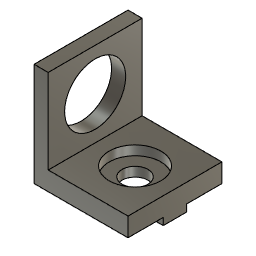
cable_holder (Autodesk Fusion 360 design; units mm, degrees)
Autodesk Fusion 360 part; units mm, degrees
sketch "Sketch1" plane through (0, 0, 0) normal (0, 0, 1) x (1, 0, 0)
  line L0 (0, 0) -> (20, 0)
  line L1 (20, 0) -> (20, 20)
  line L2 (20, 20) -> (0, 20)
  line L3 (0, 20) -> (0, 0)
  dimension "d1" = 20
  dimension "d2" = 20
  constraint horizontal L0
  constraint vertical L1
  constraint horizontal L2
  constraint vertical L3
  constraint coincident L0.start L3.end
  measures "d1" distance of L0.start L0.end
  measures "d2" distance of L0.start L2.end
extrude "Extrude1" add sketch "Sketch1" along normal blind 4
sketch "Sketch2" plane through (0, 0, 4) normal (0, 0, 1) x (-1, 0, 0)
  line L0 (0, -20) -> (0, 0)
  line L1 (0, 0) -> (-20, 0)
  line L2 (-20, 0) -> (-20, -20)
  line L3 (-20, -20) -> (0, -20)
  line L4 (-3, -20) -> (-3, 0)
  circle A0 centre (-11.5, -10) radius 2.75
  circle A1 centre (-11.5, -10) radius 5.5
  line L5 (0, -10) -> (-20, -10) construction
  dimension "d5" = 5.5
  dimension "d6" = 11
  dimension "d7" = 3
  dimension "d8" = 3
  dimension "d9" = 3
  constraint coincident L3 L4.start
  constraint coincident L1 L4.end
  constraint perpendicular L1 L4
  constraint concentric A0 A1
  constraint midpoint L0 L5.start
  constraint midpoint L2 L5.end
  constraint coincident A0.centre L5
  measures "d5" diameter of A0
  measures "d6" diameter of A1
  measures "d7" distance of L2 A1
  measures "d8" distance of L4 A1
  measures "d9" distance of L0 L4
extrude "Extrude2" cut sketch "Sketch2" against normal up to surface (4 mm away) contours A0
extrude "Extrude3" cut sketch "Sketch2" against normal blind 2 contours A1
extrude "Extrude4" add sketch "Sketch2" along normal blind 18 contours L0 L1 L3 L4
sketch "Sketch3" plane through (3, 0, 0) normal (1, 0, 0) x (0, 1, 0)
  line L0 (0, 4) -> (20, 4)
  line L1 (20, 4) -> (20, 22)
  line L2 (20, 22) -> (0, 22)
  line L3 (0, 22) -> (0, 4)
  line L4 (0, 13) -> (20, 13) construction
  line L5 (10, 22) -> (10, 4) construction
  circle A0 centre (10, 13) radius 6.5
  dimension "d16" = 13
  constraint midpoint L3 L4.start
  constraint midpoint L1 L4.end
  constraint midpoint L2 L5.start
  constraint midpoint L0 L5.end
  constraint midpoint L5 A0.centre
  measures "d16" diameter of A0
extrude "Extrude5" cut sketch "Sketch3" against normal up to surface (3 mm away) contours A0
sketch "Sketch4" plane through (0, 0, 0) normal (0, 0, -1) x (1, 0, 0)
  circle A0 centre (11.5, -10) radius 2.75
  line L0 (0, 0) -> (0, -20)
  line L1 (0, -20) -> (20, -20)
  line L2 (20, -20) -> (20, 0)
  line L3 (20, 0) -> (0, 0)
  line L4 (0, -10) -> (20, -10) construction
  line L5 (20, -12.5) -> (18.5, -12.5)
  line L6 (18.5, -12.5) -> (18.5, -7.5)
  line L7 (18.5, -7.5) -> (20, -7.5)
  line L8 (10, -20) -> (10, 0) construction
  line L9 (0, -12.5) -> (1.5, -12.5)
  line L10 (1.5, -12.5) -> (1.5, -7.5)
  line L11 (1.5, -7.5) -> (0, -7.5)
  dimension "d19" = 5
  dimension "d20" = 1.5
  dimension "d21" = 7.5
  constraint midpoint L0 L4.start
  constraint midpoint L2 L4.end
  constraint coincident L2 L5.start
  constraint perpendicular L2 L5
  constraint perpendicular L4 L6
  constraint coincident L2 L7.end
  constraint perpendicular L2 L7
  constraint midpoint L1 L8.start
  constraint midpoint L3 L8.end
  constraint symmetric L5.start L8 L9.start
  constraint symmetric L5.end L8 L9.end
  constraint symmetric L6.end L8 L10.end
  constraint symmetric L7.end L8 L11.end
  measures "d19" distance of L5.end L6.end
  measures "d20" distance of L2 L6
  measures "d21" distance of L1 L5
extrude "Extrude6" add sketch "Sketch4" along normal blind 1.5 contours L0 L9 L10 L11 | L2 L5 L6 L7
